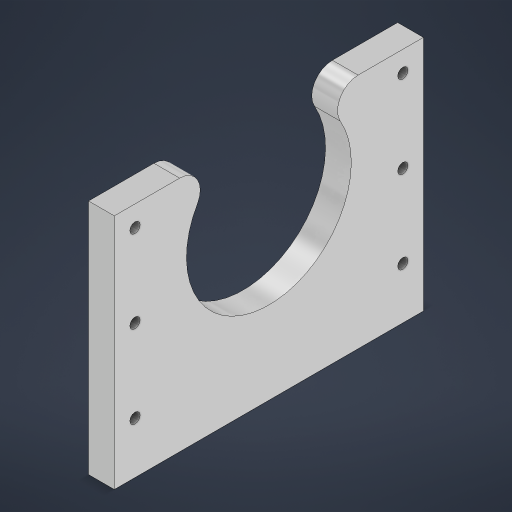
# Autodesk Inventor part: FirstStageMotorSupportPlate
Saved by Autodesk Inventor 2024 (Build 280153000, 153)
## iProperties
Created: 2024-01-05
Part Number: FirstStageMotorSupportPlate
Material: Aluminum 6061
Document SubType Name: Modeling
Designer: avsar
Density: 2.7 g/cm^3
Appearance: Aluminum - Polished
Author: avsar
Autodesk Inventor part; units mm, degrees
ref_plane "YZ Plane" through (0, 0, 0) normal (1, 0, 0) x (0, 1, 0)
ref_plane "XZ Plane" through (0, 0, 0) normal (0, 1, 0) x (-1, 0, 0)
ref_plane "XY Plane" through (0, 0, 0) normal (0, 0, 1) x (1, 0, 0)
sketch "Sketch1" plane through (0, 0, 0) normal (1, 0, 0) x (0, 1, 0)
  line L0 (-46, 60) -> (46, 60)
  line L1 (46, 60) -> (46, -60)
  line L2 (46, -60) -> (-46, -60)
  line L3 (-46, -60) -> (-46, 60)
  line L4 (-46, 60) -> (46, -60) construction
  line L5 (46, 60) -> (-46, -60) construction
  point P0 (0, 0)
  dimension "d0" = 92
  dimension "d1" = 120
  constraints: 12 end point, 2 midpoint, 2 parallel, 1 horizontal, 1 perpendicular
  measures "d0" distance of L1.end L2.end
  measures "d1" distance of L0.end L1.end
extrude "Extrusion1" add sketch "Sketch1" along normal blind 10
sketch "Sketch3" plane through (10, 0, 0) normal (1, 0, 0) x (0, 0, -1)
  circle A0 centre (0, 18) radius 32
  line L0 (-60, -46) -> (60, -46) projected
  point P0 (0, 0)
  point P1 (0, -46)
  dimension "d16" = 64
  dimension "d17" = 64
  constraints: 1 centre point, 1 midpoint, 1 vertical alignment
  measures "d16" diameter of A0
  measures "d17" distance of point (0, -46) A0.centre
extrude "Extrusion3" cut sketch "Sketch3" against normal through all
fillet "Fillet1" radius 8 2 edges at (5, 46, -15.4919) (5, 46, 15.4919)
sketch "Sketch6" plane through (0, -46, -60) normal (0, -1, 0) x (1, 0, 0)
  circle A0 centre (5, 114) radius 2
  line L0 (10, 120) -> (10, 0) construction
  circle A1 centre (5, 102) radius 2
  circle A2 centre (5, 90) radius 2
  circle A3 centre (5, 78) radius 2
  circle A4 centre (5, 66) radius 2
  circle A5 centre (5, 54) radius 2
  circle A6 centre (5, 42) radius 2
  circle A7 centre (5, 30) radius 2
  circle A8 centre (5, 18) radius 2
  circle A9 centre (5, 6) radius 2
  line L1 (5, 66) -> (5, 54) construction
  line L2 (0, 120) -> (0, 0) projected
  line L3 (0, 120) -> (10, 120) projected
  point P0 (0, 60)
  point P1 (5, 60)
  point P2 (0, 60)
  point P3 (5, 120)
  dimension "d66" = 4
  dimension "d69" = 12
  constraints: 10 centre point, 3 midpoint, 2 end point, 2 vertical, 1 horizontal alignment, 1 vertical alignment, 18 other
  measures "d66" diameter of A0
  measures "d69" distance of A0.centre A1.centre
extrude "Extrusion6" cut sketch "Sketch6" against normal blind 8
sketch "Sketch7" plane through (10, 0, 0) normal (1, 0, 0) x (0, 0, -1)
  circle A0 centre (-52, 38) radius 2
  line L0 (-34.641, 46) -> (-60, 46) construction
  line L1 (-60, 46) -> (-60, -46) construction
  line L2 (60, 46) -> (34.641, 46) construction
  line L3 (60, -46) -> (60, 46) construction
  line L4 (-60, -46) -> (60, -46) projected
  line L5 (0, 0) -> (0, -46) construction
  circle A1 centre (52, 38) radius 2
  circle A2 centre (-52, 6) radius 2
  circle A3 centre (-52, -26) radius 2
  circle A4 centre (52, 6) radius 2
  circle A5 centre (52, -26) radius 2
  dimension "d76" = 4
  dimension "d78" = 8
  dimension "d84" = 84
  dimension "d87" = 32
  constraints: 6 centre point, 3 symmetric about line, 2 end point, 1 midpoint, 1 vertical, 7 other
  measures "d76" diameter of A0
  measures "d78" distance from line of L1 A0.centre
  measures "d84" distance from line of L4 A0.centre
  measures "d87" distance of A0.centre A2.centre
extrude "Extrusion7" cut sketch "Sketch7" against normal through all
body "Solid1"
